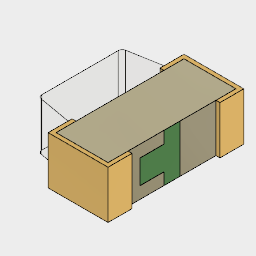
ledra_0603 (Autodesk Fusion 360 design; units mm, degrees)
Autodesk Fusion 360 part; units mm, degrees
note: some values were not read from the file. Chosen so that the rebuilt part matches the saved one: which face or edge a step refers to.
ref_plane "WorkPlane1" through (0, 0, 0.01) normal (0, 0, 1) x (1, 0, 0)
sketch "Sketch1" plane through (0, 0, 0.01) normal (0, 0, 1) x (1, 0, 0)
  line L0 (0.325, 0.8) -> (-0.325, 0.8)
  line L1 (-0.325, 0.8) -> (-0.325, -0.8)
  line L2 (-0.325, -0.8) -> (0.325, -0.8)
  line L3 (0.325, -0.8) -> (0.325, 0.8)
  line L4 (0.325, 0.8) -> (-0.325, -0.8) construction
  line L5 (-0.325, 0.8) -> (0.325, -0.8) construction
  line L6 (0, -0.8) -> (0, 0.8) construction
  line L7 (-0.375, 0.85) -> (-0.375, -0.85)
  line L8 (-0.375, -0.85) -> (0.375, -0.85)
  line L9 (0.375, -0.85) -> (0.375, 0.85)
  line L10 (0.375, 0.85) -> (-0.375, 0.85)
  line L11 (0, 0) -> (-0.7071, 0) construction
  line L12 (-0.375, -0.55) -> (-0.325, -0.55)
  line L13 (0.325, -0.55) -> (0.375, -0.55)
  line L14 (-0.375, 0.55) -> (-0.325, 0.55)
  line L15 (0.325, 0.55) -> (0.375, 0.55)
  line L16 (-0.375, 0.6) -> (-0.7837, 0.5279)
  line L17 (-0.825, 0.4787) -> (-0.825, -0.4787)
  line L18 (-0.7837, -0.5279) -> (-0.375, -0.6)
  arc A0 (-0.825, -0.4787) -> (-0.7837, -0.5279) centre (-0.775, -0.4787) ccw
  arc A1 (-0.7837, 0.5279) -> (-0.825, 0.4787) centre (-0.775, 0.4787) ccw
  dimension "d1" = 1.6
  dimension "d2" = 0.65
  dimension "d41" = 0.05
  dimension "d42" = 0.3
  dimension "d47" = 1.2
  dimension "d48" = 10
  dimension "d49" = 0.05
  dimension "d50" = 1.15
  measures "d1" distance of L0.end L1.end
  measures "d2" distance of L1.end L2.end
  measures "d42" distance of L8 L12
  measures "d47" distance of L16.start L18.end
  measures "d48" angle of L11 L18
  measures "d49" radius of A0
  measures "d50" distance of L3 L17
extrude "Extrude7" add sketch "Sketch1" along normal blind 0.6 contours L0 L1 L2 L3 makes body 1
extrude "Extrude8" add sketch "Sketch1" along normal blind 0.6 separate body contours L0 L1 L3 L7 L9 L10 L14 L15 | L1 L2 L3 L7 L8 L9 L12 L13 makes body 2 at (0.125, 0.85, 0.21) makes body 3 at (-0.125, -0.85, 0.21)
extrude "Extrude9" add sketch "Sketch1" along normal mid plane 0.6 from surface at 0.3 separate body contours L1 L7 L12 L14 | L7 L16 L17 L18 A0 A1 makes body 4
sketch "Sketch4" plane through (0.325, 0, 0) normal (1, 0, 0) x (0, 1, 0)
  line L0 (-0.8, 0.01) -> (0.8, 0.01)
  line L1 (0.8, 0.01) -> (0.8, 0.61)
  line L2 (0.8, 0.61) -> (-0.8, 0.61)
  line L3 (-0.8, 0.61) -> (-0.8, 0.01)
  line L4 (0, 0) -> (0, 0.7707) construction
  line L5 (0.1, 0.01) -> (0.1, 0.61)
  line L6 (0.1, 0.31) -> (-0.4, 0.31) construction
  line L7 (-0.4, 0.46) -> (-0.4, 0.16)
  line L8 (-0.4, 0.16) -> (-0.1, 0.16)
  line L9 (-0.1, 0.16) -> (-0.1, 0.01)
  line L10 (-0.4, 0.46) -> (-0.1, 0.46)
  line L11 (-0.1, 0.46) -> (-0.1, 0.61)
  line L12 (-0.1, 0.01) -> (0.1, 0.01)
  point P0 (0, 0.01)
  dimension "d54" = 0.2
  dimension "d55" = 0.5
  dimension "d56" = 0.3
  measures "d54" distance of L5 L9
  measures "d55" distance of L5 L7
  measures "d56" distance of L8 L10
split_face "SplitFace1" 1 faces at (0.325, -0.1833, 0.21) by curves path "Sketch4" along L11 L10 L7 L8 L9 L12 L5 on bodies 1
sketch "Sketch5" plane through (-0.325, 0, 0) normal (-1, 0, 0) x (0, -1, 0)
  line L0 (-0.8, 0.01) -> (0.8, 0.01)
  line L1 (0.8, 0.01) -> (0.8, 0.61)
  line L2 (0.8, 0.61) -> (-0.8, 0.61)
  line L3 (-0.8, 0.61) -> (-0.8, 0.01)
  line L4 (0.3, 0.21) -> (0.1, 0.21)
  line L5 (0.1, 0.21) -> (0.1, 0.41)
  line L6 (0.1, 0.41) -> (0.3, 0.41)
  line L7 (0.3, 0.41) -> (0.3, 0.21)
  line L8 (0.3, 0.21) -> (0.1, 0.41) construction
  line L9 (0.1, 0.21) -> (0.3, 0.41) construction
  line L10 (0.2, 0.01) -> (0.2, 0.61) construction
  point P0 (0.2, 0.31)
  dimension "d57" = 0.2
  dimension "d58" = 0.2
  dimension "d59" = 1
  measures "d57" distance of L5.end L6.end
  measures "d58" distance of L4.end L5.end
  measures "d59" distance of L3 P0
extrude "Extrude10" cut sketch "Sketch5" along normal blind 0.1 contours L4 L5 L6 L7 bodies 4
extrude "Extrude11" add sketch "Sketch5" along normal blind 0.1 separate body contours L4 L5 L6 L7 makes body 5
equation "d1 = ledra_0603_package_length"
equation "d2 = ledra_0603_base_width"
equation "d11 = ledra_0603_above_board"
equation "ledra_0603_package_length = 1.6 mm"
equation "ledra_0603_package_width = 1.15 mm"
equation "ledra_0603_package_height = 0.6 mm"
equation "ledra_0603_base_width = 0.65 mm"
equation "ledra_0603_lens_length = 1.2 mm"
equation "ledra_0603_lens_height = 0.6 mm"
equation "ledra_0603_above_board = 0.01 mm"
equation "ledra_0603_led_center = 1 mm"
equation "d42 = ( ledra_0603_package_length - ledra_0603_lens_length ) / 2 + 0.1 mm"
equation "d43 = ledra_0603_package_height"
equation "d45 = ledra_0603_package_height"
equation "d47 = ledra_0603_lens_length"
equation "d50 = ledra_0603_package_width"
equation "d51 = ledra_0603_package_height / 2"
equation "d52 = ledra_0603_lens_height"
equation "d56 = ledra_0603_package_height / 2"
equation "d59 = ledra_0603_led_center"
